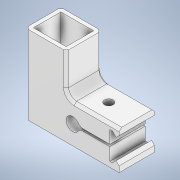
# Autodesk Inventor part: Soporte motor
Saved by Autodesk Inventor 2020.3 (Build 243373000, 373)
## iProperties
Created: 2021-04-10
Part Number: Soporte motor
Material: ABS Plastic
Document SubType Name: Modeling
Designer: juanp
Density: 1.06 g/cm^3
Appearance: Smooth - White
Author: juanp
Autodesk Inventor part; units mm, degrees
ref_plane "YZ Plane" through (0, 0, 0) normal (1, 0, 0) x (0, 1, 0)
ref_plane "XZ Plane" through (0, 0, 0) normal (0, 1, 0) x (-1, 0, 0)
ref_plane "XY Plane" through (0, 0, 0) normal (0, 0, 1) x (1, 0, 0)
sketch "Sketch1" plane through (0, 0, 0) normal (0, 1, 0) x (-1, 0, 0)
  line L0 (0, 0) -> (12.5, 0)
  line L1 (12.5, 0) -> (12.5, -10.5)
  line L2 (12.5, -10.5) -> (0, -10.5)
  line L3 (0, -10.5) -> (0, 0)
  line L4 (14, 1.5) -> (-1.5, 1.5)
  line L5 (-1.5, 1.5) -> (-1.5, -12)
  line L6 (-1.5, -12) -> (14, -12)
  line L7 (14, -12) -> (14, 1.5)
  line L8 (12.5, 0) -> (0, -10.5) construction
  circle A0 centre (6.25, -5.25) radius 1.75
  dimension "d0" = 12.5
  dimension "d1" = 10.5
  dimension "d2" = 1.5
  dimension "d3" = 1.5
  dimension "d4" = 1.5
  dimension "d5" = 1.5
  dimension "d6" = 3.5
  constraints: 18 end point, 4 parallel, 2 horizontal, 2 perpendicular, 1 centre point, 1 midpoint
  measures "d0" distance of L1.end L2.end
  measures "d1" distance of L0.end L1.end
  measures "d2" distance between parallel lines of L7 L1
  measures "d3" distance between parallel lines of L4 L0
  measures "d4" distance between parallel lines of L3 L5
  measures "d5" distance between parallel lines of L6 L2
  measures "d6" diameter of A0
extrude "Extrusion1" add sketch "Sketch1" along normal blind 1 contours L0 L1 L2 L3
extrude "Extrusion2" add sketch "Sketch1" along normal blind 30 contours L7 L6 L5 L4
sketch "Sketch2" plane through (1.5, 0, -12) normal (0, 0, -1) x (-1, 0, 0)
  line L0 (-17.6917, 12.5) -> (-16.6917, 12.5)
  line L1 (-19.0667, 11.125) -> (-17.6917, 12.5)
  line L2 (-20.1917, 12.25) -> (-19.0667, 11.125)
  line L3 (-20.1917, 2.25) -> (-20.1917, 12.25)
  line L4 (-19.0667, 3.375) -> (-20.1917, 2.25)
  line L5 (-17.6917, 2) -> (-19.0667, 3.375)
  line L6 (-16.6917, 2) -> (-17.6917, 2)
  line L7 (-16.6917, 12.5) -> (-16.6917, 2)
  line L8 (0, 0) -> (0, 0)
  line L9 (-20.1917, 2.25) -> (-20.1917, 0)
  line L10 (-20.1917, 0) -> (0, 0)
  line L11 (-20.1917, 12.25) -> (-20.1917, 14.5)
  line L12 (0, 0) -> (0, 30) projected
  line L13 (-16.6917, 7.625) -> (-4.9717, 7.625)
  line L14 (-4.9717, 6.875) -> (-16.6917, 6.875)
  line L15 (-16.6917, 6.875) -> (-16.6917, 7.625)
  line L16 (-20.1917, 14.5) -> (0, 14.5)
  arc A0 (-4.9717, 6.875) -> (-4.9717, 7.625) centre (-2.5, 7.25) ccw
  line L17 (-4.9717, 7.625) -> (-4.9717, 6.875) construction
  line L18 (0, 0) -> (0, 30) projected
  point P0 (1.5, 0)
  point P1 (-16.6917, 7.25)
  point P2 (0, 6.875)
  point P3 (0, 7)
  point P4 (0, 7.5)
  point P5 (0, 7.25)
  dimension "d11" = 0
  dimension "d12" = 3.5
  dimension "d13" = 10.5
  dimension "d14" = 90
  dimension "d15" = 90
  dimension "d16" = 10
  dimension "d17" = 1
  dimension "d18" = 45
  dimension "d19" = 45
  dimension "d25" = 0.75
  dimension "d28" = 2
  dimension "d29" = 2.5
  constraints: 34 end point, 4 point on line, 4 vertical, 3 equal length, 2 horizontal, 2 midpoint, 2 perpendicular, 2 point on circle, 1 centre point, 1 parallel, 1 tangent
  measures "d11" distance of L8.start L8.end
  measures "d12" distance between parallel lines of L3 L7
  measures "d13" distance between parallel lines of L0 L6
  measures "d14" angle of L5 L4
  measures "d15" angle of L1 L2
  measures "d16" distance of L3.start L2.start
  measures "d17" distance of L0.start L0.end
  measures "d18" angle of L3 L4
  measures "d19" angle of L2 L3
  measures "d25" distance of L13.end L14.start
  measures "d28" distance between parallel lines of L16 L0
  measures "d29" radius of A0
extrude "Extrusion3" add sketch "Sketch2" against normal up to surface (13.5 mm away) contours L1 L2 L11 L16 L12 A0 L13 L7 L0 | L14 A0 L12 L10 L9 L4 L5 L6 L7
sketch "Sketch3" plane through (1.5, 0, -12) normal (0, -1, 0) x (1, 0, 0)
  line L0 (16.6917, 0) -> (16.6917, 13.5) projected
  line L1 (16.6917, 0) -> (2.3459, 13.5) construction
  circle A0 centre (9.5188, 6.75) radius 1.65
  line L2 (-15.5, 13.5) -> (20.1917, 13.5) projected
  point P0 (11.7346, 22)
  point P1 (20.1917, 13.5)
  dimension "d22" = 3.3
  constraints: 2 end point, 1 centre point, 1 midpoint, 3 other
  measures "d22" diameter of A0
extrude "Extrusion4" cut sketch "Sketch3" against normal through all
fillet "Fillet2" radius 3 1 edges at (1.5, 14.5, -5.25)
chamfer "Chamfer1" distance 1 angle 45 8 edges at (-14, 15, -12) (-14, 15, 1.5) (1.5, 23.75, 1.5) (2.3787, 15.3787, 1.5) (13.0959, 14.5, 1.5) (1.5, 23.75, -12) (2.3787, 15.3787, -12) (13.0959, 14.5, -12)
fillet "Fillet3" radius 2.5 2 edges at (6.4717, 7.625, -5.25) (6.4717, 6.875, -5.25)
body "Solid1"
